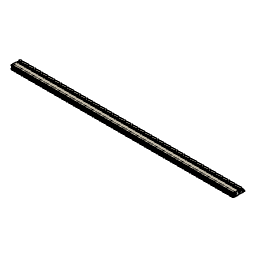
synthrotek rail profile (Autodesk Fusion 360 design; units mm, degrees)
Autodesk Fusion 360 part; units mm, degrees
sketch "Sketch1" plane through (0, 0, 0) normal (1, 0, 0) x (0, 0, -1)
  line L0 (-12.67, -4.9) -> (9.58, -4.9)
  line L1 (9.58, -4.9) -> (9.58, -3.85)
  line L2 (9.58, -3.85) -> (4.77, -3.85)
  line L3 (4.77, -3.85) -> (4.77, 2.5)
  line L4 (4.77, 2.5) -> (1.47, 2.5)
  line L5 (1.47, 2.5) -> (1.47, 1.3)
  line L6 (1.47, 1.3) -> (2.57, 1.3)
  line L7 (2.57, 1.3) -> (2.57, -1.3)
  line L8 (2.57, -1.3) -> (1.47, -1.3)
  line L9 (1.47, -1.3) -> (1.47, -2.64)
  line L10 (1.47, -2.64) -> (-1.47, -2.64)
  line L11 (-1.47, -2.64) -> (-1.47, -1.3)
  line L12 (-1.47, -1.3) -> (-2.57, -1.3)
  line L13 (-2.57, -1.3) -> (-2.57, 1.3)
  line L14 (-2.57, 1.3) -> (-1.45, 1.3)
  line L15 (-1.45, 1.3) -> (-1.45, 2.5)
  line L16 (-1.45, 2.5) -> (-12.67, 2.5)
  line L17 (-12.67, 2.5) -> (-12.67, 0.25)
  line L18 (-12.67, 0.25) -> (-10.77, 0.25)
  line L19 (-10.77, 0.25) -> (-10.77, 1.36)
  line L20 (-10.77, 1.36) -> (-8.17, 1.36)
  line L21 (-8.17, 1.36) -> (-8.17, 0.25)
  line L22 (-8.17, 0.25) -> (-6.92, 0.25)
  line L23 (-6.92, 0.25) -> (-6.92, -2.65)
  line L24 (-6.92, -2.65) -> (-8.17, -2.65)
  line L25 (-8.17, -2.65) -> (-8.17, -3.78)
  line L26 (-8.17, -3.78) -> (-10.77, -3.78)
  line L27 (-10.77, -3.78) -> (-10.77, -2.65)
  line L28 (-10.77, -2.65) -> (-12.67, -2.65)
  line L29 (-12.67, -2.65) -> (-12.67, -4.9)
  line L30 (-2.57, 0) -> (2.57, 0) construction
  line L31 (0, -2.64) -> (0, 0) construction
  circle A0 centre (0, 0) radius 2.125
  dimension "d1" = 22.25
  dimension "d2" = 1.05
  dimension "d3" = 7.4
  dimension "d4" = 3.3
  dimension "d5" = 17.44
  dimension "d6" = 11.22
  dimension "d7" = 1.14
  dimension "d8" = 2.25
  dimension "d9" = 2.25
  dimension "d10" = 5.14
  dimension "d11" = 2.6
  dimension "d12" = 5.14
  dimension "d13" = 5.75
  dimension "d14" = 2.6
  dimension "d15" = 1.9
  dimension "d16" = 1.2
  dimension "d17" = 5.14
  dimension "d18" = 2.2
  dimension "d23" = 4.25
  constraint horizontal L0
  constraint perpendicular L0 L1
  constraint perpendicular L1 L2
  constraint perpendicular L0 L3
  constraint parallel L3 L5
  constraint perpendicular L5 L6
  constraint perpendicular L6 L7
  constraint perpendicular L5 L8
  constraint perpendicular L8 L9
  constraint perpendicular L9 L10
  constraint perpendicular L10 L11
  constraint perpendicular L9 L12
  constraint perpendicular L12 L13
  constraint perpendicular L13 L14
  constraint perpendicular L12 L15
  constraint perpendicular L15 L16
  constraint perpendicular L16 L17
  constraint perpendicular L17 L18
  constraint perpendicular L18 L19
  constraint perpendicular L19 L20
  constraint perpendicular L18 L21
  constraint perpendicular L18 L23
  constraint perpendicular L23 L24
  constraint perpendicular L24 L25
  constraint perpendicular L25 L26
  constraint perpendicular L27 L28
  constraint horizontal L4
  constraint vertical L29
  constraint vertical L27
  constraint horizontal L22
  constraint collinear L17 L29
  constraint collinear L4 L16
  constraint collinear L6 L14
  constraint collinear L8 L12
  constraint collinear L21 L25
  constraint collinear L19 L27
  constraint collinear L24 L28
  constraint collinear L18 L22
  constraint equal L8 L12
  constraint collinear L5 L9
  constraint midpoint L13 L30.start
  constraint midpoint L7 L30.end
  constraint midpoint L10 L31.start
  constraint midpoint L30 L31.end
  constraint coincident L31.end A0.centre
  measures "d1" distance of L0.start L0.end
  measures "d2" distance of L0.end L1.end
  measures "d3" distance of L0 L4
  measures "d4" distance of L3.end L4.end
  measures "d5" distance of L3 L29
  measures "d6" distance of L15.end L16.end
  measures "d7" distance of L16 L20
  measures "d8" distance of L16.end L17.end
  measures "d9" distance of L0.start L28.end
  measures "d10" distance of L20 L26
  measures "d11" distance of L12.end L13.end
  measures "d12" distance of L10 L16
  measures "d13" distance of L17 L23
  measures "d14" distance of L19.end L20.end
  measures "d15" distance of L17.end L18.end
  measures "d16" distance of L14.end L15.end
  measures "d17" distance of L7 L13
  measures "d18" distance of L3 L7
  measures "d23" diameter of A0
extrude "Extrude1" add sketch "Sketch1" along normal blind 426.72 contours L0 L1 L2 L3 L4 L5 L6 L7 L8 L9 L10 L11 L12 L13 L14 L15 L16 L17 L18 L19 L20 L21 L22 L23 L24 L25 L26 L27 L28 L29 A0 | L5 L6 A0 | L14 L15 A0 | L8 L9 A0 | L11 L12 A0
extrude "Extrude2" cut sketch "Sketch1" along normal blind 2 contours L5 L6 A0 | L14 L15 A0 | L8 L9 A0 | L11 L12 A0
ref_plane "WorkPlane1" through (213.36, -1.2, 1.545) normal (1, 0, 0) x (0, 0, -1)
mirror "Mirror1" about plane through (213.36, -1.2, 1.545) normal (1, 0, 0) of "Extrude2"
equation "d9 = d8"
equation "hp_units = 84"
equation "hp_constant = 5.08 mm"
equation "d21 = hp_constant * hp_units"
